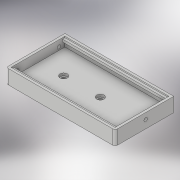
# Autodesk Inventor part: output
Saved by Autodesk Inventor 2019 (Build 230136000, 136)
## iProperties
Created: 2020-05-11
Part Number: output
Material: Generic
Document SubType Name: Modeling
Designer: Mateusz
Density: 1 g/cm^3
Appearance: Default
Author: Mateusz
Autodesk Inventor part; units mm, degrees
ref_plane "YZ Plane" through (0, 0, 0) normal (1, 0, 0) x (0, 1, 0)
ref_plane "XZ Plane" through (0, 0, 0) normal (0, 1, 0) x (-1, 0, 0)
ref_plane "XY Plane" through (0, 0, 0) normal (0, 0, 1) x (1, 0, 0)
sketch "Sketch1" plane through (0, 0, 0) normal (0, 1, 0) x (-1, 0, 0)
  line L0 (0, 0) -> (0, -44)
  line L1 (0, -44) -> (85, -44)
  line L2 (85, -44) -> (85, 0)
  line L3 (85, 0) -> (0, 0)
  line L4 (0, 2) -> (85, 2)
  line L5 (85, 2) -> (87, 2)
  line L6 (87, 2) -> (87, -44)
  line L7 (87, -44) -> (87, -46)
  line L8 (87, -46) -> (0, -46)
  line L9 (0, -46) -> (-2, -46)
  line L10 (-2, -46) -> (-2, 2)
  line L11 (-2, 2) -> (0, 2)
  dimension "d0" = 44
  dimension "d1" = 85
  dimension "d2" = 2
  dimension "d3" = 2
  dimension "d4" = 2
  dimension "d5" = 2
  constraints: 24 end point, 6 perpendicular, 4 point on line, 2 vertical
  measures "d0" distance of L0.start L0.end
  measures "d1" distance of L0.end L1.end
  measures "d2" distance of L0.start L4.start
  measures "d3" distance of L4.end L5.end
  measures "d4" distance of L6.end L7.end
  measures "d5" distance of L8.end L9.end
extrude "Extrusion1" add sketch "Sketch1" along normal blind 4 contours L3 L2 L1 L0 | L4 L5 L6 L7 L8 L9 L10 L11
extrude "Extrusion2" add sketch "Sketch1" along normal blind 10.6
sketch "Sketch2" plane through (0, 10.6, 0) normal (0, 1, 0) x (1, 0, 0)
  line L0 (-87, -2) -> (-87, 46) projected
  line L1 (-87, -2) -> (-87, 46)
  line L2 (2, 46) -> (2, -2) projected
  line L3 (-87, 46) -> (2, 46)
  line L4 (2, 46) -> (2, -2)
  line L5 (2, -2) -> (-87, -2)
  line L6 (-85, 44) -> (-85, 0) projected
  line L7 (-85, 0) -> (-85, 44)
  line L8 (-85, 44) -> (0, 44)
  line L9 (0, 44) -> (0, 0) projected
  line L10 (0, 44) -> (0, 0)
  line L11 (0, 0) -> (-85, 0)
  line L12 (-85, 0) -> (-85, 2)
  line L13 (-85, 2) -> (0, 2)
  line L14 (-85, 44) -> (-85, 42)
  line L15 (-85, 42) -> (0, 42)
  dimension "d10" = 2
  dimension "d11" = 2
  constraints: 24 end point, 5 perpendicular, 4 point on line, 3 collinear, 1 parallel, 1 vertical
  measures "d10" distance of L6.end L12.end
  measures "d11" distance of L6.start L14.end
extrude "Extrusion3" add sketch "Sketch2" against normal blind 2 contours L8 L9 L15 L6 | L13 L9 L11 L6
extrude "Extrusion4" add sketch "Sketch2" along normal blind 1
fillet "Fillet1" radius 2 1 edges at (2, 5.8, 2)
sketch "Sketch3" plane through (2, 0, -46) normal (1, 0, 0) x (0, 0, -1)
  line L0 (0, 11.6) -> (-46, 11.6) projected
  line L1 (-23, 11.6) -> (-23, 6.6)
  circle A0 centre (-23, 6.6) radius 1.45
  point P0 (-46, 0)
  dimension "d17" = 5
  dimension "d18" = 2.9
  constraints: 2 end point, 1 centre point, 1 coincident, 1 midpoint, 1 vertical
  measures "d17" distance of L1.start L1.end
  measures "d18" diameter of A0
extrude "Extrusion5" cut sketch "Sketch3" against normal blind 15
sketch "Sketch4" plane through (-87, 0, -46) normal (-1, 0, 0) x (0, 0, 1)
  line L0 (46, 11.6) -> (0, 11.6) projected
  line L1 (0, 11.6) -> (2, 11.6)
  line L2 (2, 11.6) -> (7, 11.6)
  line L3 (7, 11.6) -> (7, 6.6)
  line L4 (46, 0) -> (46, 11.6) projected
  line L5 (46, 11.6) -> (41, 11.6)
  line L6 (2, 11.6) -> (46, 11.6) projected
  line L7 (41, 11.6) -> (41, 6.6)
  circle A0 centre (7, 6.6) radius 1.45
  circle A1 centre (41, 6.6) radius 1.45
  dimension "d21" = 2
  dimension "d22" = 5
  dimension "d23" = 5
  dimension "d24" = 5
  dimension "d25" = 5
  dimension "d26" = 2.9
  dimension "d27" = 2.9
  constraints: 10 end point, 3 point on line, 2 centre point, 2 coincident, 2 perpendicular
  measures "d21" distance of L0.end L1.end
  measures "d22" distance of L1.end L2.end
  measures "d23" distance of L2.end L3.end
  measures "d24" distance of L0.start L5.end
  measures "d25" distance of L5.end L7.end
  measures "d26" diameter of A0
  measures "d27" diameter of A1
extrude "Extrusion6" cut sketch "Sketch4" against normal blind 15
sketch "Sketch5" plane through (0, 4, 0) normal (0, 1, 0) x (1, 0, 0)
  line L0 (-87, 46) -> (-87, 0) projected
  line L1 (-87, 23) -> (-65, 23)
  line L2 (-65, 23) -> (-35, 23)
  circle A0 centre (-65, 23) radius 1.65
  circle A1 centre (-35, 23) radius 1.65
  circle A2 centre (-35, 23) radius 3
  circle A3 centre (-65, 23) radius 3
  point P0 (0, 0)
  dimension "d30" = 22
  dimension "d31" = 30
  dimension "d32" = 3.3
  dimension "d33" = 3.3
  dimension "d34" = 6
  dimension "d35" = 6
  constraints: 4 centre point, 4 coincident, 4 end point, 2 horizontal, 1 midpoint
  measures "d30" distance of L1.start L1.end
  measures "d31" distance of L1.end L2.end
  measures "d32" diameter of A0
  measures "d33" diameter of A1
  measures "d34" diameter of A2
  measures "d35" diameter of A3
extrude "Extrusion7" cut sketch "Sketch5" against normal blind 10 contours A1 | A0 L2 L1 | L1 L2 A0
extrude "Extrusion8" cut sketch "Sketch5" against normal blind 2 contours A3 L2 A0 L1 | A2 | L1 A0 L2 A3
body "Solid1"
